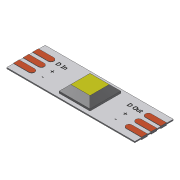
# Autodesk Inventor part: LED_einzel
Saved by Autodesk Inventor 2021.3 (Build 253353000, 353)
## iProperties
Part Number: LED_einzel
Material: Generisch
Document SubType Name: Modeling
Designer: fanki
Density: 1 g/cm^3
Appearance: Vorgabe
Mass: 0.208903 g
Surface Area: 7.46482 cm^2
Volume: 0.208903 cm^3
ROT_Weight: 0.209 g
ROT_Weight_Num: 0.00020890288934415134
Author: fanki
Autodesk Inventor part; units mm, degrees
ref_plane "YZ Plane" through (0, 0, 0) normal (1, 0, 0) x (0, 1, 0)
ref_plane "XZ Plane" through (0, 0, 0) normal (0, 1, 0) x (-1, 0, 0)
ref_plane "XY Plane" through (0, 0, 0) normal (0, 0, 1) x (1, 0, 0)
sketch "Skizze1" plane through (0, 0, 0) normal (0, 0, 1) x (1, 0, 0)
  line L0 (-16.665, 5) -> (16.665, 5)
  line L1 (16.665, 5) -> (16.665, -5)
  line L2 (16.665, -5) -> (-16.665, -5)
  line L3 (-16.665, -5) -> (-16.665, 5)
  point P0 (0, 0)
  point P1 (-16.665, 0)
  point P2 (0, 5)
  dimension "d0" = 33.33
  dimension "d1" = 16.665
  dimension "d2" = 10
  constraints: 8 end point, 2 midpoint, 2 parallel, 1 horizontal, 1 horizontal alignment, 1 perpendicular
  measures "d0" distance of L0.start L0.end
  measures "d1" distance from line of L3 point (0, 0)
  measures "d2" distance of L2.end L0.start
extrude "Extrusion1" add sketch "Skizze1" along normal blind 0.3
sketch "Skizze2" plane through (0, 0, 0.3) normal (0, 0, 1) x (1, 0, 0)
  line L0 (-4, 4) -> (4, 4)
  line L1 (4, 4) -> (4, -4)
  line L2 (4, -4) -> (-4, -4)
  line L3 (-4, -4) -> (-4, 4)
  point P0 (0, 0)
  dimension "d5" = 8
  dimension "d6" = 8
  dimension "d7" = 4
  dimension "d8" = 4
  constraints: 8 end point, 2 parallel, 1 horizontal, 1 perpendicular
  measures "d5" distance of L0.start L0.end
  measures "d6" distance of L2.end L0.start
  measures "d7" distance from line of point (0, 0) L0
  measures "d8" distance from line of point (0, 0) L1
extrude "Extrusion2" add sketch "Skizze2" along normal blind 2
chamfer "Fase1" distance 1.5 angle 45 4 edges at (0, 4, 2.3) (4, 0, 2.3) (-4, 0, 2.3) (0, -4, 2.3)
sketch "Skizze3" plane through (0, 0, 0.3) normal (0, 0, 1) x (1, 0, 0)
  line L0 (-16.665, 0.75) -> (-12.665, 0.75)
  line L1 (-12.665, 0.75) -> (-12.665, -0.75)
  line L2 (-12.665, -0.75) -> (-16.665, -0.75)
  line L3 (-16.665, -0.75) -> (-16.665, 0.75)
  line L4 (16.665, -5) -> (16.665, 5) projected
  line L5 (16.665, -4.247) -> (12.665, -4.247)
  line L6 (12.665, -4.247) -> (12.665, -2.747)
  line L7 (12.665, -2.747) -> (16.665, -2.747)
  line L8 (16.665, -2.747) -> (16.665, -4.247)
  line L9 (16.5002, -0.75) -> (12.665, -0.75)
  line L10 (12.665, -0.75) -> (12.665, 0.75)
  line L11 (12.665, 0.75) -> (16.5002, 0.75)
  line L12 (16.5002, 0.75) -> (16.5002, -0.75)
  line L13 (16.665, 2.25) -> (12.665, 2.25)
  line L14 (12.665, 2.25) -> (12.665, 3.75)
  line L15 (12.665, 3.75) -> (16.665, 3.75)
  line L16 (16.665, 3.75) -> (16.665, 2.25)
  arc A0 (-12.665, -0.75) -> (-12.665, 0.75) centre (-12.665, 0) ccw
  line L17 (-16.665, 5) -> (-16.665, -5) projected
  line L18 (-16.665, 3.25) -> (-12.665, 3.25)
  line L19 (-16.665, 1.75) -> (-16.665, 3.25)
  line L20 (-12.665, 1.75) -> (-16.665, 1.75)
  arc A1 (-12.665, 1.75) -> (-12.665, 3.25) centre (-12.665, 2.5) ccw
  line L21 (-16.665, -1.75) -> (-12.665, -1.75)
  line L22 (-16.665, -3.25) -> (-16.665, -1.75)
  line L23 (-12.665, -3.25) -> (-16.665, -3.25)
  arc A2 (-12.665, -3.25) -> (-12.665, -1.75) centre (-12.665, -2.5) ccw
  line L24 (-16.665, 0.75) -> (-12.665, 0.75)
  line L25 (-16.665, -0.75) -> (-16.665, 0.75)
  line L26 (-12.665, -0.75) -> (-16.665, -0.75)
  arc A3 (-12.665, -0.75) -> (-12.665, 0.75) centre (-12.665, 0) ccw
  point P0 (0, 0)
  point P1 (-16.665, 0)
  point P2 (-16.665, 0)
  point P3 (-16.665, 0)
  point P4 (-16.665, 2.5)
  point P5 (-16.665, -2.5)
  point P6 (-16.665, 0)
  dimension "d14" = 1.5
  dimension "d18" = 4
  dimension "d21" = 2.5
  dimension "d24" = 2.5
  constraints: 50 end point, 8 parallel, 8 point on circle, 4 centre point, 4 collinear, 4 horizontal, 4 perpendicular, 3 midpoint, 3 point on line, 2 vertical, 1 coincident, 1 horizontal alignment, 1 tangent, 30 other
  measures "d14" distance of L0.end L1.end
  measures "d18" distance of L0.start L0.end
  measures "d21" distance of L0.start L18.start
  measures "d24" distance of L0.start L21.start
extrude "Extrusion3" add sketch "Skizze3" along normal blind 0.1 contours L0 L1 L2 L3 | A0 L1 | L18 A1 L20 L17 | L21 A2 L23 L17
mirror "Spiegeln1" about plane through (0, 0, 0) normal (1, 0, 0) of "Extrusion3"
sketch "Skizze4" plane through (0, 0, 0.3) normal (0, 0, 1) x (1, 0, 0)
  line L0 (-12.2968, 3.2694) -> (-7.2917, 3.2694) construction
  line L1 (-7.2917, 3.2694) -> (-7.2917, 1.7306) construction
  line L2 (-7.2917, 1.7306) -> (-12.2968, 1.7306) construction
  line L3 (-12.2968, 1.7306) -> (-12.2968, 3.2694) construction
  line L4 (-16.665, 3.25) -> (-16.665, 1.75) projected
  line L5 (6.6813, 3.3311) -> (11.6865, 3.3311) construction
  line L6 (11.6865, 3.3311) -> (11.6865, 1.7923) construction
  line L7 (11.6865, 1.7923) -> (6.6813, 1.7923) construction
  line L8 (6.6813, 1.7923) -> (6.6813, 3.3311) construction
  line L9 (-12.1976, -1.7306) -> (-7.3909, -1.7306) construction
  line L10 (-7.3909, -1.7306) -> (-7.3909, -3.2694) construction
  line L11 (-7.3909, -3.2694) -> (-12.1976, -3.2694) construction
  line L12 (-12.1976, -3.2694) -> (-12.1976, -1.7306) construction
  line L13 (-12.2968, 0.7694) -> (-7.2917, 0.7694) construction
  line L14 (-7.2917, 0.7694) -> (-7.2917, -0.7694) construction
  line L15 (-7.2917, -0.7694) -> (-12.2968, -0.7694) construction
  line L16 (-12.2968, -0.7694) -> (-12.2968, 0.7694) construction
  line L17 (6.6813, -1.7306) -> (11.6865, -1.7306) construction
  line L18 (11.6865, -1.7306) -> (11.6865, -3.2694) construction
  line L19 (11.6865, -3.2694) -> (6.6813, -3.2694) construction
  line L20 (6.6813, -3.2694) -> (6.6813, -1.7306) construction
  line L21 (6.6813, 0.7694) -> (11.6865, 0.7694) construction
  line L22 (11.6865, 0.7694) -> (11.6865, -0.7694) construction
  line L23 (11.6865, -0.7694) -> (6.6813, -0.7694) construction
  line L24 (6.6813, -0.7694) -> (6.6813, 0.7694) construction
  line L25 (-16.665, 0.75) -> (-16.665, -0.75) projected
  line L26 (-16.665, -1.75) -> (-16.665, -3.25) projected
  line L27 (16.665, 0.75) -> (16.665, -0.75) projected
  line L28 (16.665, -1.75) -> (16.665, -3.25) projected
  arc A0 (12.665, 3.25) -> (12.665, 1.75) centre (12.665, 2.5) ccw projected
  line L29 (16.665, 3.25) -> (16.665, 1.75) projected
  line L30 (12.665, -1.75) -> (16.665, -1.75) projected
  line L31 (16.665, -1.75) -> (16.665, -0.75) projected
  line L32 (16.665, -0.75) -> (12.665, -0.75) projected
  arc A1 (12.665, 0.75) -> (12.665, -0.75) centre (12.665, 0) ccw projected
  line L33 (12.665, 0.75) -> (16.665, 0.75) projected
  line L34 (16.665, 0.75) -> (16.665, 1.75) projected
  line L35 (16.665, 1.75) -> (12.665, 1.75) projected
  arc A2 (12.665, 3.25) -> (12.665, 1.75) centre (12.665, 2.5) ccw projected
  line L36 (12.665, 3.25) -> (16.665, 3.25) projected
  line L37 (16.665, 3.25) -> (16.665, 5) projected
  line L38 (16.665, 5) -> (-16.665, 5) projected
  line L39 (-16.665, 5) -> (-16.665, 3.25) projected
  line L40 (-16.665, 3.25) -> (-12.665, 3.25) projected
  arc A3 (-12.665, 1.75) -> (-12.665, 3.25) centre (-12.665, 2.5) ccw projected
  line L41 (-12.665, 1.75) -> (-16.665, 1.75) projected
  line L42 (-16.665, 1.75) -> (-16.665, 0.75) projected
  line L43 (-16.665, 0.75) -> (-12.665, 0.75) projected
  arc A4 (-12.665, -0.75) -> (-12.665, 0.75) centre (-12.665, 0) ccw projected
  line L44 (-12.665, -0.75) -> (-16.665, -0.75) projected
  line L45 (-16.665, -0.75) -> (-16.665, -1.75) projected
  line L46 (-16.665, -1.75) -> (-12.665, -1.75) projected
  arc A5 (-12.665, -3.25) -> (-12.665, -1.75) centre (-12.665, -2.5) ccw projected
  line L47 (-12.665, -3.25) -> (-16.665, -3.25) projected
  line L48 (-16.665, -3.25) -> (-16.665, -5) projected
  line L49 (-16.665, -5) -> (16.665, -5) projected
  line L50 (16.665, -5) -> (16.665, -3.25) projected
  line L51 (16.665, -3.25) -> (12.665, -3.25) projected
  arc A6 (12.665, -1.75) -> (12.665, -3.25) centre (12.665, -2.5) ccw projected
  line L52 (4, 4) -> (4, -4) projected
  line L53 (4, -4) -> (-4, -4) projected
  line L54 (-4, -4) -> (-4, 4) projected
  line L55 (-4, 4) -> (4, 4) projected
  spline S0 degree 2 poles (-10.2254, 2.4992) (-10.2254, 2.3622) (-10.3364, 2.1418) (-10.4296, 2.0802) knots 0 0 0 1 2 2 2
  spline S1 degree 2 poles (-10.4296, 2.0802) (-10.5058, 2.0324) (-10.6622, 2) (-10.7837, 2) knots 0 0 0 1 2 2 2
  line L56 (-10.7837, 2) -> (-11.0139, 2)
  line L57 (-11.0139, 2) -> (-11.0139, 3)
  line L58 (-11.0139, 3) -> (-10.7861, 3)
  spline S2 degree 2 poles (-10.7861, 3) (-10.6451, 3) (-10.4847, 2.9579) (-10.428, 2.9206) knots 0 0 0 1 2 2 2
  spline S3 degree 2 poles (-10.428, 2.9206) (-10.3315, 2.8566) (-10.2254, 2.6451) (-10.2254, 2.4992) knots 0 0 0 1 2 2 2
  spline S4 degree 2 poles (-10.3639, 2.5008) (-10.3639, 2.6159) (-10.4401, 2.7788) (-10.5155, 2.825) knots 0 0 0 1 2 2 2
  spline S5 degree 2 poles (-10.5155, 2.825) (-10.569, 2.8566) (-10.6897, 2.8849) (-10.7797, 2.8849) knots 0 0 0 1 2 2 2
  line L59 (-10.7797, 2.8849) -> (-10.881, 2.8849)
  line L60 (-10.881, 2.8849) -> (-10.881, 2.1151)
  line L61 (-10.881, 2.1151) -> (-10.7797, 2.1151)
  spline S6 degree 2 poles (-10.7797, 2.1151) (-10.6913, 2.1151) (-10.5576, 2.1434) (-10.5033, 2.1815) knots 0 0 0 1 2 2 2
  spline S7 degree 2 poles (-10.5033, 2.1815) (-10.4336, 2.2285) (-10.3639, 2.3841) (-10.3639, 2.5008) knots 0 0 0 1 2 2 2
  line L62 (-9.3032, 2) -> (-9.6905, 2)
  line L63 (-9.6905, 2) -> (-9.6905, 2.1021)
  line L64 (-9.6905, 2.1021) -> (-9.5633, 2.1021)
  line L65 (-9.5633, 2.1021) -> (-9.5633, 2.8979)
  line L66 (-9.5633, 2.8979) -> (-9.6905, 2.8979)
  line L67 (-9.6905, 2.8979) -> (-9.6905, 3)
  line L68 (-9.6905, 3) -> (-9.3032, 3)
  line L69 (-9.3032, 3) -> (-9.3032, 2.8979)
  line L70 (-9.3032, 2.8979) -> (-9.4304, 2.8979)
  line L71 (-9.4304, 2.8979) -> (-9.4304, 2.1021)
  line L72 (-9.4304, 2.1021) -> (-9.3032, 2.1021)
  line L73 (-9.3032, 2.1021) -> (-9.3032, 2)
  line L74 (-8.5592, 2) -> (-8.6857, 2)
  line L75 (-8.6857, 2) -> (-8.6857, 2.4279)
  spline S8 degree 2 poles (-8.6857, 2.4279) (-8.6857, 2.4797) (-8.6954, 2.5689) (-8.71, 2.5956) knots 0 0 0 1 2 2 2
  spline S9 degree 2 poles (-8.71, 2.5956) (-8.7254, 2.624) (-8.7805, 2.6515) (-8.8275, 2.6515) knots 0 0 0 1 2 2 2
  spline S10 degree 2 poles (-8.8275, 2.6515) (-8.8745, 2.6515) (-8.9741, 2.6013) (-9.022, 2.5608) knots 0 0 0 1 2 2 2
  line L76 (-9.022, 2.5608) -> (-9.022, 2)
  line L77 (-9.022, 2) -> (-9.1484, 2)
  line L78 (-9.1484, 2) -> (-9.1484, 2.7504)
  line L79 (-9.1484, 2.7504) -> (-9.022, 2.7504)
  line L80 (-9.022, 2.7504) -> (-9.022, 2.6669)
  spline S11 degree 2 poles (-9.022, 2.6669) (-8.9652, 2.718) (-8.8558, 2.7715) (-8.7942, 2.7715) knots 0 0 0 1 2 2 2
  spline S12 degree 2 poles (-8.7942, 2.7715) (-8.684, 2.7715) (-8.5592, 2.6256) (-8.5592, 2.487) knots 0 0 0 1 2 2 2
  line L81 (-8.5592, 2.487) -> (-8.5592, 2)
  line L82 (-9.3992, -0.0539) -> (-9.7379, -0.0539)
  line L83 (-9.7379, -0.0539) -> (-9.7379, -0.3926)
  line L84 (-9.7379, -0.3926) -> (-9.8498, -0.3926)
  line L85 (-9.8498, -0.3926) -> (-9.8498, -0.0539)
  line L86 (-9.8498, -0.0539) -> (-10.1885, -0.0539)
  line L87 (-10.1885, -0.0539) -> (-10.1885, 0.0539)
  line L88 (-10.1885, 0.0539) -> (-9.8498, 0.0539)
  line L89 (-9.8498, 0.0539) -> (-9.8498, 0.3926)
  line L90 (-9.8498, 0.3926) -> (-9.7379, 0.3926)
  line L91 (-9.7379, 0.3926) -> (-9.7379, 0.0539)
  line L92 (-9.7379, 0.0539) -> (-9.3992, 0.0539)
  line L93 (-9.3992, 0.0539) -> (-9.3992, -0.0539)
  line L94 (-9.6046, -2.5608) -> (-9.9831, -2.5608)
  line L95 (-9.9831, -2.5608) -> (-9.9831, -2.4392)
  line L96 (-9.9831, -2.4392) -> (-9.6046, -2.4392)
  line L97 (-9.6046, -2.4392) -> (-9.6046, -2.5608)
  spline S13 degree 2 poles (8.2925, 2.5609) (8.2925, 2.4239) (8.1815, 2.2035) (8.0883, 2.1419) knots 0 0 0 1 2 2 2
  spline S14 degree 2 poles (8.0883, 2.1419) (8.0121, 2.0941) (7.8557, 2.0617) (7.7341, 2.0617) knots 0 0 0 1 2 2 2
  line L98 (7.7341, 2.0617) -> (7.504, 2.0617)
  line L99 (7.504, 2.0617) -> (7.504, 3.0617)
  line L100 (7.504, 3.0617) -> (7.7317, 3.0617)
  spline S15 degree 2 poles (7.7317, 3.0617) (7.8727, 3.0617) (8.0332, 3.0195) (8.0899, 2.9823) knots 0 0 0 1 2 2 2
  spline S16 degree 2 poles (8.0899, 2.9823) (8.1863, 2.9182) (8.2925, 2.7067) (8.2925, 2.5609) knots 0 0 0 1 2 2 2
  spline S17 degree 2 poles (8.1539, 2.5625) (8.1539, 2.6776) (8.0777, 2.8405) (8.0024, 2.8866) knots 0 0 0 1 2 2 2
  spline S18 degree 2 poles (8.0024, 2.8866) (7.9489, 2.9182) (7.8282, 2.9466) (7.7382, 2.9466) knots 0 0 0 1 2 2 2
  line L101 (7.7382, 2.9466) -> (7.6369, 2.9466)
  line L102 (7.6369, 2.9466) -> (7.6369, 2.1768)
  line L103 (7.6369, 2.1768) -> (7.7382, 2.1768)
  spline S19 degree 2 poles (7.7382, 2.1768) (7.8265, 2.1768) (7.9602, 2.2051) (8.0145, 2.2432) knots 0 0 0 1 2 2 2
  spline S20 degree 2 poles (8.0145, 2.2432) (8.0842, 2.2902) (8.1539, 2.4458) (8.1539, 2.5625) knots 0 0 0 1 2 2 2
  spline S21 degree 2 poles (9.5737, 2.9474) (9.6304, 2.881) (9.6936, 2.6865) (9.6936, 2.5617) knots 0 0 0 1 2 2 2
  spline S22 degree 2 poles (9.6936, 2.5617) (9.6936, 2.4401) (9.632, 2.2432) (9.5737, 2.1768) knots 0 0 0 1 2 2 2
  spline S23 degree 2 poles (9.5737, 2.1768) (9.5121, 2.1071) (9.3492, 2.0406) (9.2512, 2.0406) knots 0 0 0 1 2 2 2
  spline S24 degree 2 poles (9.2512, 2.0406) (9.1499, 2.0406) (8.9878, 2.1095) (8.9286, 2.1768) knots 0 0 0 1 2 2 2
  spline S25 degree 2 poles (8.9286, 2.1768) (8.8711, 2.2432) (8.8095, 2.4385) (8.8095, 2.5617) knots 0 0 0 1 2 2 2
  spline S26 degree 2 poles (8.8095, 2.5617) (8.8095, 2.6873) (8.8719, 2.8785) (8.9294, 2.9474) knots 0 0 0 1 2 2 2
  spline S27 degree 2 poles (8.9294, 2.9474) (8.9878, 3.0139) (9.1507, 3.0828) (9.2512, 3.0828) knots 0 0 0 1 2 2 2
  spline S28 degree 2 poles (9.2512, 3.0828) (9.3533, 3.0828) (9.517, 3.0114) (9.5737, 2.9474) knots 0 0 0 1 2 2 2
  spline S29 degree 2 poles (9.5551, 2.5617) (9.5551, 2.6605) (9.5121, 2.8137) (9.4732, 2.864) knots 0 0 0 1 2 2 2
  spline S30 degree 2 poles (9.4732, 2.864) (9.4335, 2.9158) (9.3217, 2.9677) (9.252, 2.9677) knots 0 0 0 1 2 2 2
  spline S31 degree 2 poles (9.252, 2.9677) (9.1799, 2.9677) (9.0713, 2.9174) (9.0299, 2.864) knots 0 0 0 1 2 2 2
  spline S32 degree 2 poles (9.0299, 2.864) (8.9902, 2.8129) (8.9481, 2.6589) (8.9481, 2.5617) knots 0 0 0 1 2 2 2
  spline S33 degree 2 poles (8.9481, 2.5617) (8.9481, 2.3648) (9.1134, 2.1557) (9.252, 2.1557) knots 0 0 0 1 2 2 2
  spline S34 degree 2 poles (9.252, 2.1557) (9.3905, 2.1557) (9.5551, 2.3648) (9.5551, 2.5617) knots 0 0 0 1 2 2 2
  line L104 (10.4132, 2.0617) -> (10.2868, 2.0617)
  line L105 (10.2868, 2.0617) -> (10.2868, 2.1443)
  spline S35 degree 2 poles (10.2868, 2.1443) (10.2285, 2.0933) (10.1239, 2.0406) (10.0591, 2.0406) knots 0 0 0 1 2 2 2
  spline S36 degree 2 poles (10.0591, 2.0406) (10.0105, 2.0406) (9.9238, 2.073) (9.8922, 2.1079) knots 0 0 0 1 2 2 2
  spline S37 degree 2 poles (9.8922, 2.1079) (9.8598, 2.1427) (9.8241, 2.2489) (9.8241, 2.3251) knots 0 0 0 1 2 2 2
  line L106 (9.8241, 2.3251) -> (9.8241, 2.8121)
  line L107 (9.8241, 2.8121) -> (9.9505, 2.8121)
  line L108 (9.9505, 2.8121) -> (9.9505, 2.3842)
  spline S38 degree 2 poles (9.9505, 2.3842) (9.9505, 2.3242) (9.9594, 2.2456) (9.9748, 2.2165) knots 0 0 0 1 2 2 2
  spline S39 degree 2 poles (9.9748, 2.2165) (9.9902, 2.1873) (10.0429, 2.1605) (10.0923, 2.1605) knots 0 0 0 1 2 2 2
  spline S40 degree 2 poles (10.0923, 2.1605) (10.1385, 2.1605) (10.2431, 2.2132) (10.2868, 2.2513) knots 0 0 0 1 2 2 2
  line L109 (10.2868, 2.2513) -> (10.2868, 2.8121)
  line L110 (10.2868, 2.8121) -> (10.4132, 2.8121)
  line L111 (10.4132, 2.8121) -> (10.4132, 2.0617)
  spline S41 degree 2 poles (10.8233, 2.0471) (10.7204, 2.0471) (10.6045, 2.1646) (10.6045, 2.2918) knots 0 0 0 1 2 2 2
  line L112 (10.6045, 2.2918) -> (10.6045, 2.7076)
  line L113 (10.6045, 2.7076) -> (10.5194, 2.7076)
  line L114 (10.5194, 2.7076) -> (10.5194, 2.8121)
  line L115 (10.5194, 2.8121) -> (10.6045, 2.8121)
  line L116 (10.6045, 2.8121) -> (10.6045, 3.0276)
  line L117 (10.6045, 3.0276) -> (10.7309, 3.0276)
  line L118 (10.7309, 3.0276) -> (10.7309, 2.8121)
  line L119 (10.7309, 2.8121) -> (10.9635, 2.8121)
  line L120 (10.9635, 2.8121) -> (10.9635, 2.7076)
  line L121 (10.9635, 2.7076) -> (10.7309, 2.7076)
  line L122 (10.7309, 2.7076) -> (10.7309, 2.3502)
  spline S42 degree 2 poles (10.7309, 2.3502) (10.7309, 2.2934) (10.735, 2.2311) (10.7487, 2.2043) knots 0 0 0 1 2 2 2
  spline S43 degree 2 poles (10.7487, 2.2043) (10.7601, 2.1808) (10.8111, 2.1573) (10.8549, 2.1573) knots 0 0 0 1 2 2 2
  spline S44 degree 2 poles (10.8549, 2.1573) (10.8857, 2.1573) (10.9432, 2.1759) (10.9562, 2.1816) knots 0 0 0 1 2 2 2
  line L123 (10.9562, 2.1816) -> (10.9635, 2.1816)
  line L124 (10.9635, 2.1816) -> (10.9635, 2.0682)
  spline S45 degree 2 poles (10.9635, 2.0682) (10.9278, 2.0584) (10.8549, 2.0471) (10.8233, 2.0471) knots 0 0 0 1 2 2 2
  line L125 (9.579, -0.0539) -> (9.2402, -0.0539)
  line L126 (9.2402, -0.0539) -> (9.2402, -0.3926)
  line L127 (9.2402, -0.3926) -> (9.1284, -0.3926)
  line L128 (9.1284, -0.3926) -> (9.1284, -0.0539)
  line L129 (9.1284, -0.0539) -> (8.7897, -0.0539)
  line L130 (8.7897, -0.0539) -> (8.7897, 0.0539)
  line L131 (8.7897, 0.0539) -> (9.1284, 0.0539)
  line L132 (9.1284, 0.0539) -> (9.1284, 0.3926)
  line L133 (9.1284, 0.3926) -> (9.2402, 0.3926)
  line L134 (9.2402, 0.3926) -> (9.2402, 0.0539)
  line L135 (9.2402, 0.0539) -> (9.579, 0.0539)
  line L136 (9.579, 0.0539) -> (9.579, -0.0539)
  line L137 (9.3735, -2.5608) -> (8.9951, -2.5608)
  line L138 (8.9951, -2.5608) -> (8.9951, -2.4392)
  line L139 (8.9951, -2.4392) -> (9.3735, -2.4392)
  line L140 (9.3735, -2.4392) -> (9.3735, -2.5608)
  point P0 (0, 0)
  point P1 (-7.2917, 2.5)
  point P2 (-16.665, 2.5)
  point P3 (11.6865, 2.5617)
  point P4 (-7.3909, -2.5)
  point P5 (-7.2917, 0)
  point P6 (11.6865, -2.5)
  point P7 (11.6865, 0)
  point P8 (-16.665, 0)
  point P9 (-16.665, -2.5)
  point P10 (16.665, 0)
  point P11 (16.665, -2.5)
  point P12 (11.915, 2.5)
  point P13 (16.665, 2.5)
  point P14 (9.1839, -1.7306)
  point P15 (9.1839, -0.7694)
  point P16 (9.1839, 0.7694)
  point P17 (9.1839, 1.7923)
  point P18 (-9.7942, 1.7306)
  point P19 (-9.7942, 0.7694)
  point P20 (-9.7942, -0.7694)
  point P21 (-9.7942, -1.7306)
  constraints: 20 midpoint, 6 horizontal alignment, 4 vertical alignment, 1 point on circle, 12 other
emboss "Prägen1" sketch "Skizze4" operation add depth 0.01 direction (0, 0, -1) contours S0 S1 L56 L57 L58 S2 S3 | L62 L63 L64 L65 L66 L67 L68 L69 L70 L71 L72 L73 | L74 L75 S8 S9 S10 L76 L77 L78 L79 L80 S11 S12 L81 | L82 L83 L84 L85 L86 L87 L88 L89 L90 L91 L92 L93 | L94 L95 L96 L97 | S13 S14 L98 L99 L100 S15 S16 | S21 S22 S23 S24 S25 S26 S27 S28 | L104 L105 S35 S36 S37 L106 L107 L108 S38 S39 S40 L109 L110 L111 | S41 L112 L113 L114 L115 L116 L117 L118 L119 L120 L121 L122 S42 S43 S44 L123 L124 S45 | L125 L126 L127 L128 L129 L130 L131 L132 L133 L134 L135 L136 | L137 L138 L139 L140
sketch "Skizze5" plane through (0, 0, 0) normal (0, 0, -1) x (-1, 0, 0)
  line L0 (12.665, -1.75) -> (16.665, -1.75) projected
  line L1 (16.665, -1.75) -> (16.665, -3.25) projected
  line L2 (16.665, -3.25) -> (12.665, -3.25) projected
  arc A0 (12.665, -1.75) -> (12.665, -3.25) centre (12.665, -2.5) ccw projected
  line L3 (12.665, 0.75) -> (16.665, 0.75) projected
  line L4 (16.665, 0.75) -> (16.665, -0.75) projected
  line L5 (16.665, -0.75) -> (12.665, -0.75) projected
  arc A1 (12.665, 0.75) -> (12.665, -0.75) centre (12.665, 0) ccw projected
  line L6 (12.665, 3.25) -> (16.665, 3.25) projected
  line L7 (16.665, 3.25) -> (16.665, 1.75) projected
  line L8 (16.665, 1.75) -> (12.665, 1.75) projected
  arc A2 (12.665, 3.25) -> (12.665, 1.75) centre (12.665, 2.5) ccw projected
  line L9 (-12.665, 3.25) -> (-16.665, 3.25) projected
  arc A3 (-12.665, 1.75) -> (-12.665, 3.25) centre (-12.665, 2.5) ccw projected
  line L10 (-16.665, 1.75) -> (-12.665, 1.75) projected
  line L11 (-16.665, 3.25) -> (-16.665, 1.75) projected
  line L12 (-12.665, 0.75) -> (-16.665, 0.75) projected
  arc A4 (-12.665, -0.75) -> (-12.665, 0.75) centre (-12.665, 0) ccw projected
  line L13 (-16.665, -0.75) -> (-12.665, -0.75) projected
  line L14 (-16.665, 0.75) -> (-16.665, -0.75) projected
  line L15 (-12.665, -1.75) -> (-16.665, -1.75) projected
  arc A5 (-12.665, -3.25) -> (-12.665, -1.75) centre (-12.665, -2.5) ccw projected
  line L16 (-16.665, -3.25) -> (-12.665, -3.25) projected
  line L17 (-16.665, -1.75) -> (-16.665, -3.25) projected
  point P0 (0, 0)
extrude "Extrusion4" add sketch "Skizze5" along normal blind 0.2
equation "\"d1\" = 0.5 * d0"
equation "\"d7\" = 0.5 * d6"
equation "\"d8\" = 0.5 * d5"
